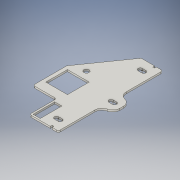
# Autodesk Inventor part: gantry inner
Saved by Autodesk Inventor 2018.2 (Build 222227000, 227)
## iProperties
Created: 2017-12-18
Part Number: gantry inner
Material: Steel
Document SubType Name: Modeling
Designer: torba
Density: 7.85 g/cm^3
Appearance: Steel
Author: torba
Autodesk Inventor part; units mm, degrees
ref_plane "YZ Plane" through (0, 0, 0) normal (1, 0, 0) x (0, 1, 0)
ref_plane "XZ Plane" through (0, 0, 0) normal (0, 1, 0) x (-1, 0, 0)
ref_plane "XY Plane" through (0, 0, 0) normal (0, 0, 1) x (1, 0, 0)
sketch "Sketch1" plane through (0, 0, 0) normal (0, 1, 0) x (-1, 0, 0)
  line L0 (0, 0) -> (184.15, 0)
  line L1 (184.15, 0) -> (184.15, -368.3)
  line L2 (184.15, -368.3) -> (0, -368.3)
  line L3 (0, -368.3) -> (0, 0)
  line L4 (171.45, -127) -> (94.742, -127)
  line L5 (94.742, -127) -> (94.742, -203.708)
  line L6 (94.742, -203.708) -> (171.45, -203.708)
  line L7 (171.45, -203.708) -> (171.45, -127)
  line L8 (95.25, -6.35) -> (69.85, -6.35)
  line L9 (69.85, -6.35) -> (69.85, -82.55)
  line L10 (69.85, -82.55) -> (95.25, -82.55)
  line L11 (95.25, -82.55) -> (95.25, -6.35)
  line L12 (184.15, -82.55) -> (101.6, -82.55)
  line L13 (101.6, -82.55) -> (101.6, 0)
  line L14 (184.15, -192.6167) -> (184.15, -218.0167)
  line L15 (101.6, -82.55) -> (101.6, -368.3) construction
  line L16 (0, 0) -> (0, -184.15)
  line L17 (0, 0) -> (19.05, 0)
  line L18 (19.05, 0) -> (19.05, -368.3) construction
  line L19 (19.05, -368.3) -> (0, -368.3)
  line L20 (0, -368.3) -> (0, 0)
  line L21 (19.05, -368.3) -> (19.05, -331.75) construction
  line L22 (19.05, 0) -> (19.05, -36.55) construction
  line L23 (19.05, -36.55) -> (36.55, -36.55) construction
  line L24 (19.05, -331.75) -> (36.55, -331.75) construction
  circle A0 centre (36.55, -36.55) radius 17.5 construction
  circle A1 centre (36.55, -331.75) radius 17.5 construction
  line L25 (19.05, -184.15) -> (-7.975, -184.15) construction
  circle A2 centre (-7.975, -184.15) radius 18.6165 construction
  line L26 (0, -166.65) -> (0, -141.25)
  line L27 (0, -201.65) -> (0, -227.05)
  line L28 (0, -141.25) -> (0, -115.85)
  line L29 (0, -227.05) -> (0, -252.45)
  line L30 (0, -214.35) -> (0, -153.95)
  circle A3 centre (-7.975, -184.15) radius 7.5
  circle A4 centre (36.55, -331.75) radius 7.5
  circle A5 centre (36.55, -36.55) radius 7.5
  line L31 (-26.5915, -184.15) -> (-39.2915, -184.15) construction
  line L32 (-39.2915, -184.15) -> (-39.2915, -202.7665)
  line L33 (-39.2915, -184.15) -> (-39.2915, -165.5335)
  line L34 (-39.2915, -165.5335) -> (16.2751, -165.5335) construction
  line L35 (-39.2915, -202.7665) -> (16.2751, -202.7665) construction
  line L36 (0, 0) -> (0, -126.2421)
  line L37 (0, -368.3) -> (0, -223.0079)
  line L38 (-7.975, -202.7665) -> (-7.975, -215.4665) construction
  line L39 (-7.975, -165.5335) -> (-7.975, -152.8335) construction
  line L40 (0, -152.8335) -> (-39.2915, -152.8335)
  line L41 (-39.2915, -152.8335) -> (-39.2915, -215.4665)
  line L42 (-39.2915, -215.4665) -> (0, -215.4665)
  line L43 (0, -215.4665) -> (0, -152.8335)
  line L44 (0, -368.3) -> (76.2, -368.3)
  line L45 (76.2, -368.3) -> (184.15, -368.3)
  line L46 (184.15, -191.77) -> (184.15, -213.8739)
  line L47 (184.15, -213.8739) -> (76.2, -368.3)
  line L48 (184.15, -190.5) -> (184.15, -213.8739)
  line L49 (184.15, -82.55) -> (101.6, -82.55)
  line L50 (101.6, -82.55) -> (101.6, -95.25)
  line L51 (101.6, -95.25) -> (184.15, -95.25)
  line L52 (184.15, -95.25) -> (184.15, -82.55)
  dimension "d0" = 184.15
  dimension "d1" = 368.3
  dimension "d7" = 25.4
  dimension "d8" = 76.2
  dimension "d13" = 44.45
  dimension "d15" = 82.55
  dimension "d16" = 76.708
  dimension "d17" = 6.35
  dimension "d18" = 0
  dimension "d22" = 19.05
  dimension "d23" = 36.55
  dimension "d24" = 36.55
  dimension "d25" = 17.5
  dimension "d26" = 17.5
  dimension "d27" = 6.35
  dimension "d28" = 27.025
  dimension "d38" = 15
  dimension "d39" = 15
  dimension "d43" = 12.7
  dimension "d46" = 12.7
  dimension "d47" = 12.7
  dimension "d56" = 76.2
  dimension "d60" = 37.2329
  dimension "d61" = 15
  dimension "d62" = 58.3415
  dimension "d63" = 58.3415
  dimension "d64" = 31.3165
  dimension "d65" = 31.3165
  dimension "d66" = 2.775
  dimension "d67" = 2.775
  dimension "d68" = 68.3
  dimension "d69" = 57.9079
  dimension "d70" = 42.9
  dimension "d71" = 30.2
  dimension "d72" = 17.5
  dimension "d73" = 30.2
  dimension "d74" = 42.9
  dimension "d75" = 68.3
  dimension "d82" = 76.708
  dimension "d85" = 110.0667
  dimension "d86" = 135.4667
  dimension "d87" = 140.4579
  dimension "d99" = 12.7
  dimension "d101" = 10.1659
  dimension "d116" = 12.7
  constraints: 106 end point, 24 point on line, 14 horizontal, 12 parallel, 11 perpendicular, 6 coincident, 5 centre point, 3 collinear, 3 midpoint, 3 point on circle, 3 tangent, 1 horizontal alignment, 1 vertical, 2 other
  measures "d0" distance of L1.end L2.end
  measures "d1" distance of L0.end L1.end
  measures "d7" distance of L10.end L9.end
  measures "d8" distance of L9.end L8.end
  measures "d13" distance between parallel lines of L4 L12
  measures "d15" distance of L12.start L12.end
  measures "d16" distance between parallel lines of L6 L4
  measures "d17" distance between parallel lines of L11 L13
  measures "d18" distance between parallel lines of L12 L10
  measures "d22" distance of L18.end L19.end
  measures "d23" distance of L18.end L21.end
  measures "d24" distance of L17.end L22.end
  measures "d25" distance of L22.end L23.end
  measures "d26" distance of L21.end L24.end
  measures "d27" distance between parallel lines of L8 L0
  measures "d28" distance of L25.start L25.end
  measures "d38" diameter of A4
  measures "d39" diameter of A5
  measures "d43" distance of L31.start L31.end
  measures "d46" distance of L38.start L38.end
  measures "d47" distance of L39.start L39.end
  measures "d56" distance of L19.end L44.end
  measures "d60" diameter of A2
  measures "d61" diameter of A3
  measures "d62" distance between parallel lines of L18 L33
  measures "d63" distance between parallel lines of L18 L41
  measures "d64" distance between parallel lines of L25 L40
  measures "d65" distance between parallel lines of L42 L25
  measures "d66" distance from line of L34.end L18
  measures "d67" distance from line of L35.end L18
  measures "d68" distance from line of L28.end L25
  measures "d69" distance from line of L36.end L25
  measures "d70" distance from line of L26.end L25
  measures "d71" distance from line of L30.end L25
  measures "d72" distance from line of L27.start L25
  measures "d73" distance from line of L30.start L25
  measures "d74" distance from line of L27.end L25
  measures "d75" distance from line of L29.end L25
  measures "d82" distance between parallel lines of L5 L7
  measures "d85" distance from line of L14.start L12
  measures "d86" distance from line of L14.end L12
  measures "d87" distance from line of L37.end L12
  measures "d99" distance between parallel lines of L1 L7
  measures "d101" distance from line of L6 L46.end
  measures "d116" distance of L50.end L49.end
extrude "Extrusion3" add sketch "Sketch1" along normal blind 6.35 contours L0 L13 L50 L51 L1 L47 L2 L3 | L12 L1 L51 L50 | L3 L42 L41 L32 L33 L40 | L1 L2 L47
extrude "Extrusion4" cut sketch "Sketch1" along normal blind 25.4 contours L12 L1 L51 L50 | L1 L2 L47
fillet "Fillet1" radius 25.4 4 edges at (39.2915, 3.175, -152.8335) (39.2915, 3.175, -215.4665) (0, 3.175, -215.4665) (0, 3.175, -152.8335)
fillet "Fillet4" radius 6.35 7 edges at (-101.6, 3.175, 0) (0, 3.175, 0) (0, 3.175, -368.3) (-184.15, 3.175, -213.8739) (-76.2, 3.175, -368.3) (-184.15, 3.175, -95.25) (-101.6, 3.175, -95.25)
sketch "Sketch2" plane through (0, 6.35, 0) normal (0, 1, 0) x (1, 0, 0)
  arc A0 (0, 361.95) -> (-6.35, 368.3) centre (-6.35, 361.95) ccw projected
  line L0 (-6.35, 368.3) -> (-72.8912, 368.3) projected
  line L1 (-78.0957, 365.5881) -> (-183.0045, 215.5126) projected
  line L2 (-184.15, 211.8745) -> (-184.15, 101.6) projected
  arc A1 (-101.6, 6.35) -> (-95.25, 0) centre (-95.25, 6.35) ccw projected
  line L3 (-95.25, 0) -> (-6.35, 0) projected
  arc A2 (-6.35, 0) -> (0, 6.35) centre (-6.35, 6.35) ccw projected
  line L4 (0, 6.35) -> (0, 128.7543) projected
  arc A3 (19.6457, 153.4939) -> (39.2915, 178.2335) centre (13.8915, 178.2335) ccw projected
  line L5 (39.2915, 178.2335) -> (39.2915, 190.0665) projected
  arc A4 (39.2915, 190.0665) -> (19.6457, 214.8061) centre (13.8915, 190.0665) ccw projected
  line L6 (0, 239.5457) -> (0, 361.95) projected
  line L7 (-171.45, 127) -> (-171.45, 203.708) projected
  line L8 (-171.45, 203.708) -> (-94.742, 203.708) projected
  line L9 (-94.742, 203.708) -> (-94.742, 127) projected
  line L10 (-94.742, 127) -> (-171.45, 127) projected
  line L11 (-95.25, 6.35) -> (-95.25, 82.55) projected
  line L12 (-95.25, 82.55) -> (-69.85, 82.55) projected
  line L13 (-69.85, 82.55) -> (-69.85, 6.35) projected
  line L14 (-69.85, 6.35) -> (-95.25, 6.35) projected
  circle A5 centre (-36.55, 36.55) radius 7.5 projected
  circle A6 centre (-36.55, 331.75) radius 7.5 projected
  circle A7 centre (7.975, 184.15) radius 7.5 projected
  line L15 (-30.2, 36.55) -> (-42.9, 36.55) construction
  line L16 (-30.2, 44.05) -> (-42.9, 44.05)
  line L17 (-42.9, 29.05) -> (-30.2, 29.05)
  arc A8 (-30.2, 29.05) -> (-30.2, 44.05) centre (-30.2, 36.55) ccw
  arc A9 (-42.9, 44.05) -> (-42.9, 29.05) centre (-42.9, 36.55) ccw
  line L18 (14.325, 184.15) -> (1.625, 184.15) construction
  line L19 (14.325, 191.65) -> (1.625, 191.65)
  line L20 (1.625, 176.65) -> (14.325, 176.65)
  arc A10 (14.325, 176.65) -> (14.325, 191.65) centre (14.325, 184.15) ccw
  arc A11 (1.625, 191.65) -> (1.625, 176.65) centre (1.625, 184.15) ccw
  line L21 (-30.2, 331.75) -> (-42.9, 331.75) construction
  circle A12 centre (-36.55, 331.75) radius 7.5 projected
  line L22 (-30.2, 339.25) -> (-42.9, 339.25)
  line L23 (-42.9, 324.25) -> (-30.2, 324.25)
  arc A13 (-30.2, 324.25) -> (-30.2, 339.25) centre (-30.2, 331.75) ccw
  arc A14 (-42.9, 339.25) -> (-42.9, 324.25) centre (-42.9, 331.75) ccw
  arc A15 (-72.8912, 368.3) -> (-78.0957, 365.5881) centre (-72.8912, 361.95) ccw projected
  arc A16 (-183.0045, 215.5126) -> (-184.15, 211.8745) centre (-177.8, 211.8745) ccw projected
  arc A17 (19.6457, 153.4939) -> (0, 128.7543) centre (25.4, 128.7543) ccw projected
  arc A18 (0, 239.5457) -> (19.6457, 214.8061) centre (25.4, 239.5457) ccw projected
  line L24 (-177.8, 95.25) -> (-107.95, 95.25) projected
  line L25 (-101.6, 88.9) -> (-101.6, 6.35) projected
  arc A19 (-184.15, 101.6) -> (-177.8, 95.25) centre (-177.8, 101.6) ccw projected
  arc A20 (-101.6, 88.9) -> (-107.95, 95.25) centre (-107.95, 88.9) ccw projected
  point P0 (0, 0)
  dimension "d91" = 6.35
  dimension "d92" = 15
  dimension "d93" = 6.35
  dimension "d94" = 15
  dimension "d95" = 6.35
  dimension "d96" = 15
  constraints: 24 end point, 12 point on circle, 12 tangent, 6 centre point, 5 parallel, 3 midpoint, 1 horizontal
  measures "d91" distance of A5.centre L15.end
  measures "d92" diameter of A9
  measures "d93" distance of A7.centre L18.end
  measures "d94" diameter of A11
  measures "d95" distance of A12.centre L21.end
  measures "d96" diameter of A14
extrude "Extrusion5" cut sketch "Sketch2" against normal blind 25.4 contours A5 L16 A8 L17 | A5 L17 A9 L16 | A6 L22 A13 L23 | A6 L23 A14 L22 | A7 L19 A10 L20 | A7 L20 A11 L19
sketch "Sketch4" plane through (0, 6.35, 0) normal (0, 1, 0) x (1, 0, 0)
  line L0 (-30.2, 29.05) -> (-42.9, 29.05) projected
  line L1 (-42.9, 44.05) -> (-30.2, 44.05) projected
  line L2 (1.625, 191.65) -> (14.325, 191.65) projected
  line L3 (14.325, 176.65) -> (1.625, 176.65) projected
  line L4 (-42.9, 339.25) -> (-30.2, 339.25) projected
  line L5 (-30.2, 324.25) -> (-42.9, 324.25) projected
  line L6 (-36.55, 339.25) -> (-36.55, 324.25)
  line L7 (7.975, 191.65) -> (7.975, 176.65)
  line L8 (-36.55, 44.05) -> (-36.55, 29.05)
  circle A0 centre (-36.55, 36.55) radius 1.27
  circle A1 centre (7.975, 184.15) radius 1.27
  circle A2 centre (-36.55, 331.75) radius 1.27
  point P0 (0, 0)
  dimension "d103" = 2.54
  dimension "d104" = 2.54
  dimension "d105" = 2.54
  constraints: 9 midpoint, 6 end point, 3 centre point
  measures "d103" diameter of A0
  measures "d104" diameter of A1
  measures "d105" diameter of A2
extrude "Extrusion6" add sketch "Sketch4" against normal up to surface (6.35 mm away) separate body
sketch "Sketch6" plane through (-95.25, 0, 0) normal (0, 0, 1) x (1, 0, 0)
  line L0 (22.3588, 6.35) -> (22.3588, 0) projected
  line L1 (88.9, 6.35) -> (88.9, 0) projected
  line L2 (0, 6.35) -> (88.9, 6.35) projected
  line L3 (0, 0) -> (0, 6.35) projected
  line L4 (0, 0) -> (88.9, 0) projected
  line L5 (0, 6.35) -> (88.9, 6.35) projected
  line L6 (88.9, 6.35) -> (73.025, 6.35)
  line L7 (73.025, 6.35) -> (66.675, 6.35)
  line L8 (66.675, 6.35) -> (66.675, 0)
  line L9 (66.675, 0) -> (73.025, 0)
  line L10 (73.025, 0) -> (73.025, 6.35)
  point P0 (95.25, 0)
  dimension "d108" = 15.875
  dimension "d109" = 6.35
  dimension "d110" = 6.35
  constraints: 10 end point, 2 parallel, 1 horizontal, 1 perpendicular, 1 point on line
  measures "d108" distance of L1.start L6.end
  measures "d109" distance of L9.end L8.end
  measures "d110" distance of L8.end L7.end
extrude "Extrusion7" cut sketch "Sketch6" against normal blind 6.35 contours L2 L10 L4 L8 bodies 1
sketch "Sketch8" plane through (-6.35, 0, -368.3) normal (0, 0, -1) x (-1, 0, 0)
  line L0 (15.875, 6.35) -> (15.875, 0) projected
  line L1 (22.225, 0) -> (22.225, 6.35) projected
  line L2 (22.225, 6.35) -> (15.875, 6.35) projected
  line L3 (15.875, 0) -> (22.225, 0) projected
  point P0 (-6.35, 0)
extrude "Extrusion8" cut sketch "Sketch8" against normal blind 6.35 bodies 1
sketch "Sketch9" plane through (0, 0, 0) normal (0, -1, 0) x (1, 0, 0)
  line L0 (-22.225, -361.95) -> (-22.225, -368.3) projected
  line L1 (-6.35, -368.3) -> (-22.225, -368.3) projected
  arc A0 (-6.35, -368.3) -> (0, -361.95) centre (-6.35, -361.95) ccw projected
  line L2 (0, -239.5457) -> (0, -361.95) projected
  arc A1 (19.6457, -214.8061) -> (0, -239.5457) centre (25.4, -239.5457) ccw projected
  arc A2 (19.6457, -214.8061) -> (39.2915, -190.0665) centre (13.8915, -190.0665) ccw projected
  line L3 (39.2915, -178.2335) -> (39.2915, -190.0665) projected
  arc A3 (39.2915, -178.2335) -> (19.6457, -153.4939) centre (13.8915, -178.2335) ccw projected
  arc A4 (0, -128.7543) -> (19.6457, -153.4939) centre (25.4, -128.7543) ccw projected
  line L4 (0, -6.35) -> (0, -128.7543) projected
  arc A5 (0, -6.35) -> (-6.35, 0) centre (-6.35, -6.35) ccw projected
  line L5 (-22.225, 0) -> (-6.35, 0) projected
  line L6 (-22.225, 0) -> (-22.225, -6.35) projected
  line L7 (-22.225, -6.35) -> (-28.575, -6.35) projected
  line L8 (-28.575, -6.35) -> (-28.575, 0) projected
  line L9 (-95.25, 0) -> (-28.575, 0) projected
  arc A6 (-95.25, 0) -> (-101.6, -6.35) centre (-95.25, -6.35) ccw projected
  line L10 (-101.6, -6.35) -> (-101.6, -88.9) projected
  arc A7 (-107.95, -95.25) -> (-101.6, -88.9) centre (-107.95, -88.9) ccw projected
  line L11 (-107.95, -95.25) -> (-177.8, -95.25) projected
  arc A8 (-177.8, -95.25) -> (-184.15, -101.6) centre (-177.8, -101.6) ccw projected
  line L12 (-184.15, -211.8745) -> (-184.15, -101.6) projected
  arc A9 (-184.15, -211.8745) -> (-183.0045, -215.5126) centre (-177.8, -211.8745) ccw projected
  line L13 (-183.0045, -215.5126) -> (-78.0957, -365.5881) projected
  arc A10 (-78.0957, -365.5881) -> (-72.8912, -368.3) centre (-72.8912, -361.95) ccw projected
  line L14 (-28.575, -368.3) -> (-72.8912, -368.3) projected
  line L15 (-28.575, -368.3) -> (-28.575, -361.95) projected
  line L16 (-28.575, -361.95) -> (-22.225, -361.95) projected
  line L17 (-42.9, -324.25) -> (-30.2, -324.25) projected
  arc A11 (-30.2, -339.25) -> (-30.2, -324.25) centre (-30.2, -331.75) ccw projected
  line L18 (-30.2, -339.25) -> (-42.9, -339.25) projected
  arc A12 (-42.9, -324.25) -> (-42.9, -339.25) centre (-42.9, -331.75) ccw projected
  line L19 (-42.9, -29.05) -> (-30.2, -29.05) projected
  arc A13 (-30.2, -44.05) -> (-30.2, -29.05) centre (-30.2, -36.55) ccw projected
  line L20 (-30.2, -44.05) -> (-42.9, -44.05) projected
  arc A14 (-42.9, -29.05) -> (-42.9, -44.05) centre (-42.9, -36.55) ccw projected
  line L21 (1.625, -176.65) -> (14.325, -176.65) projected
  arc A15 (14.325, -191.65) -> (14.325, -176.65) centre (14.325, -184.15) ccw projected
  line L22 (14.325, -191.65) -> (1.625, -191.65) projected
  arc A16 (1.625, -176.65) -> (1.625, -191.65) centre (1.625, -184.15) ccw projected
  line L23 (-171.45, -203.708) -> (-171.45, -127) projected
  line L24 (-171.45, -127) -> (-94.742, -127) projected
  line L25 (-94.742, -127) -> (-94.742, -203.708) projected
  line L26 (-94.742, -203.708) -> (-171.45, -203.708) projected
  line L27 (-95.25, -82.55) -> (-95.25, -6.35) projected
  line L28 (-95.25, -6.35) -> (-69.85, -6.35) projected
  line L29 (-69.85, -6.35) -> (-69.85, -82.55) projected
  line L30 (-69.85, -82.55) -> (-95.25, -82.55) projected
  line L31 (-94.742, -127) -> (-94.742, -203.708) projected
  line L32 (-94.742, -203.708) -> (-94.742, -232.283)
  line L33 (-94.742, -232.283) -> (-133.096, -232.283)
  point P0 (0, 0)
  dimension "d117" = 28.575
  dimension "d125" = 38.354
  constraints: 4 end point, 2 coincident, 1 horizontal, 1 vertical
  measures "d117" distance of L25.end L32.end
  measures "d125" distance of L33.start L33.end
hole "Hole2" at (-133.096, 0, -232.283) direction (0, 1, 0) diameter 18.161 depth 25.4 tip angle 118 bodies 1
equation "\"d24\" = d23"
equation "\"d26\" = d25"
body "Solid2"
body "Solid3"
